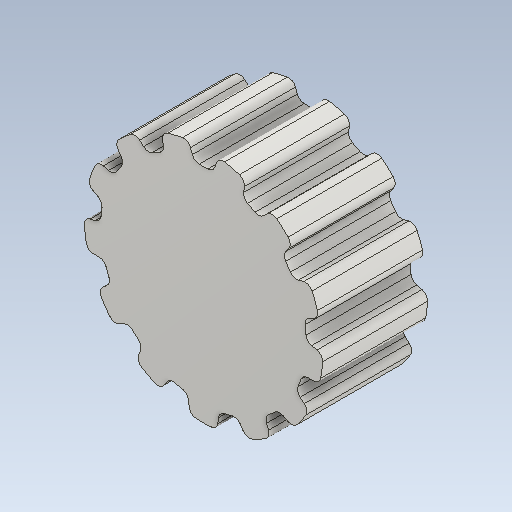
# Autodesk Inventor part: Синхронный шкив3
Saved by Autodesk Inventor 2021 (Build 250183000, 183)
## iProperties
Created: 2021-06-15
Part Number: Синхронный шкив3
Material: Steel
Document SubType Name: Modeling
Designer: panda
Density: 1 g/cm^3
Appearance: Steel
CustomPartVersion: 1
Author: panda
Autodesk Inventor part; units mm, degrees
ref_plane "YZ Plane" through (0, 0, 0) normal (1, 0, 0) x (0, 1, 0)
ref_plane "XZ Plane" through (0, 0, 0) normal (0, 1, 0) x (-1, 0, 0)
ref_plane "XY Plane" through (0, 0, 0) normal (0, 0, 1) x (1, 0, 0)
sketch "Эскиз шкива" plane through (0, 0, 0) normal (0, 0, 1) x (1, 0, 0)
  circle A0 centre (0, 0) radius 19.7074 construction
  circle A1 centre (0, 0) radius 19.3264
  circle A2 centre (0, 0) radius 16.6594
  line L0 (-2.4385, 19.1719) -> (-1.524, 16.6594)
  line L1 (-1.524, 16.6594) -> (1.524, 16.6594)
  line L2 (1.524, 16.6594) -> (2.4385, 19.1719)
  line L3 (0, 0) -> (0, 19.3264) construction
  point P0 (0, 16.6594)
  dimension "d0" = 39.4147
  dimension "d1" = 0.381
  dimension "d2" = 2.667
  dimension "d3" = 40
  dimension "d4" = 3.048
  constraints: 8 end point, 3 coincident, 3 point on circle, 2 centre point, 1 horizontal, 1 midpoint, 1 point on line, 1 vertical, 1 vertical alignment, 3 other
  measures "d0" diameter of A0
  measures "d1" radial gap between concentric circles of A0 A1
  measures "d3" angle of L2 L0
  measures "d4" distance of L0.end L1.end
extrude "Базовое тело" add sketch "Эскиз шкива" along normal mid plane 17.018 contours A2 | A1 L0 L1 L2 | L2 L1 L0 A1
extrude "Зуб" cut sketch "Эскиз шкива" along normal through all both and the other way through all contours L2 L1 L0 A1 picked at (0, 18.4259)
fillet "Fillet" radius 1.1938 2 edges at (1.524, 16.6594, 0) (-1.524, 16.6594, 0)
fillet "Fillet" radius 1.1684 4 edges at (-2.4385, 19.1719, 4.2545) (-2.4385, 19.1719, -4.2545) (2.4385, 19.1719, 4.2545) (2.4385, 19.1719, -4.2545)
pattern_circular "Зубья" count 13 over 360 about axis through (0, 0, -10) along (0, 0, 1) of "Зуб", "Fillet"
feature "Левый фланец" [suppressed]
feature "Правый фланец" [suppressed]
equation "\"d1\" = da_a"
equation "\"d2\" = da_hg"
equation "\"d3\" = 2 * da_fi"
equation "\"d4\" = da_bw"
equation "\"d5\" = da_bf"
equation "\"d7\" = da_bf"
equation "\"d9\" = da_rb"
equation "\"d10\" = da_rt"
equation "\"da_pb\" = 9.525"
equation "\"da_fi\" = 20deg"
equation "\"da_hg\" = 2.667"
equation "\"da_bw\" = 3.048"
equation "\"da_rb\" = 1.1938"
equation "\"da_rt\" = 1.1684"
equation "\"da_a\" = 0.381"
equation "\"da_bf\" = 17.018"
equation "\"da_wf\" = 1.5"
equation "\"da_hf\" = 1.5"
body "Solid1"
